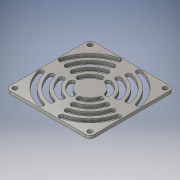
# Autodesk Inventor part: Lüftergitter
Saved by Autodesk Inventor 2016 (Build 200138000, 138)
## iProperties
Created: 2018-05-17
Part Number: Lüftergitter
Material: Stainless Steel
Document SubType Name: Modeling
Designer: Phil Erle
Density: 8 g/cm^3
Appearance: Semi-Polished
Author: Phil Erle
Autodesk Inventor part; units mm, degrees
ref_plane "YZ Plane" through (0, 0, 0) normal (1, 0, 0) x (0, 1, 0)
ref_plane "XZ Plane" through (0, 0, 0) normal (0, 1, 0) x (-1, 0, 0)
ref_plane "XY Plane" through (0, 0, 0) normal (0, 0, 1) x (1, 0, 0)
sketch "Sketch1" plane through (0, 0, 0) normal (0, 0, 1) x (1, 0, 0)
  line L0 (-40, -40) -> (40, -40)
  line L1 (40, -40) -> (40, 40)
  line L2 (40, 40) -> (-40, 40)
  line L3 (-40, 40) -> (-40, -40)
  line L4 (-40, -40) -> (40, 40) construction
  line L5 (40, -40) -> (-40, 40) construction
  point P0 (0, 0)
  dimension "d0" = 80
  dimension "d1" = 80
  constraints: 12 end point, 2 midpoint, 2 parallel, 1 horizontal, 1 perpendicular
  measures "d0" distance of L1.end L2.end
  measures "d1" distance of L0.end L1.end
extrude "Extrusion1" add sketch "Sketch1" along normal blind 3
sketch "Sketch2" plane through (0, 0, 3) normal (0, 0, 1) x (1, 0, 0)
  arc A0 (-9.8351, 36.7052) -> (-36.7052, 9.8351) centre (0, 0) ccw construction
  arc A1 (-10.4822, 39.12) -> (-39.12, 10.4822) centre (0, 0) ccw
  arc A2 (-9.1881, 34.2904) -> (-34.2904, 9.1881) centre (0, 0) ccw
  arc A3 (-9.1881, 34.2904) -> (-10.4822, 39.12) centre (-9.8351, 36.7052) ccw
  arc A4 (-39.12, 10.4822) -> (-34.2904, 9.1881) centre (-36.7052, 9.8351) ccw
  arc A5 (-7.7646, 28.9778) -> (-28.9778, 7.7646) centre (0, 0) ccw construction
  arc A6 (-8.4116, 31.3926) -> (-31.3926, 8.4116) centre (0, 0) ccw
  arc A7 (-7.1175, 26.563) -> (-26.563, 7.1175) centre (0, 0) ccw
  arc A8 (-7.1175, 26.563) -> (-8.4116, 31.3926) centre (-7.7646, 28.9778) ccw
  arc A9 (-31.3926, 8.4116) -> (-26.563, 7.1175) centre (-28.9778, 7.7646) ccw
  arc A10 (-5.694, 21.2504) -> (-21.2504, 5.694) centre (0, 0) ccw construction
  arc A11 (-6.3411, 23.6652) -> (-23.6652, 6.3411) centre (0, 0) ccw
  arc A12 (-5.047, 18.8356) -> (-18.8356, 5.047) centre (0, 0) ccw
  arc A13 (-5.047, 18.8356) -> (-6.3411, 23.6652) centre (-5.694, 21.2504) ccw
  arc A14 (-23.6652, 6.3411) -> (-18.8356, 5.047) centre (-21.2504, 5.694) ccw
  line L0 (0, 0) -> (-62.4866, 0) construction
  line L1 (0, 0) -> (-61.1079, 16.3738) construction
  line L2 (0, 0) -> (0, 46.5462) construction
  line L3 (0, 0) -> (-12.1401, 45.3074) construction
  arc A15 (-3.6235, 13.523) -> (-13.523, 3.6235) centre (0, 0) ccw construction
  arc A16 (-4.2705, 15.9378) -> (-15.9378, 4.2705) centre (0, 0) ccw
  arc A17 (-2.9764, 11.1081) -> (-11.1081, 2.9764) centre (0, 0) ccw
  arc A18 (-2.9764, 11.1081) -> (-4.2705, 15.9378) centre (-3.6235, 13.523) ccw
  arc A19 (-15.9378, 4.2705) -> (-11.1081, 2.9764) centre (-13.523, 3.6235) ccw
  dimension "d4" = 38
  dimension "d5" = 15
  dimension "d6" = 15
  dimension "d7" = 30
  dimension "d8" = 22
  dimension "d9" = 5
  dimension "d10" = 5
  dimension "d11" = 5
  dimension "d12" = 14
  dimension "d13" = 5
  constraints: 40 point on circle, 20 centre point, 16 tangent, 8 end point, 8 point on line, 4 coincident, 1 horizontal, 1 vertical
  measures "d4" radius of A0
  measures "d5" angle of L0 L1
  measures "d6" angle of L3 L2
  measures "d7" radius of A5
  measures "d8" radius of A10
  measures "d9" radial gap between concentric circles of A2 A1
  measures "d10" radial gap between concentric circles of A7 A6
  measures "d11" radial gap between concentric circles of A12 A11
  measures "d12" radius of A15
  measures "d13" diameter of A18
extrude "Extrusion2" cut sketch "Sketch2" against normal blind 3
pattern_circular "Circular Pattern1" count 4 over 360 about axis through (0, 0, -10) along (0, 0, 1) of "Extrusion2"
sketch "Sketch3" plane through (0, 0, 3) normal (0, 0, 1) x (1, 0, 0)
  line L0 (-35.75, -35.75) -> (35.75, -35.75) construction
  line L1 (35.75, -35.75) -> (35.75, 35.75) construction
  line L2 (35.75, 35.75) -> (-35.75, 35.75) construction
  line L3 (-35.75, 35.75) -> (-35.75, -35.75) construction
  line L4 (-35.75, -35.75) -> (35.75, 35.75) construction
  line L5 (35.75, -35.75) -> (-35.75, 35.75) construction
  point P0 (0, 0)
  dimension "d19" = 71.5
  dimension "d20" = 71.5
  constraints: 12 end point, 4 coincident, 2 midpoint, 2 parallel, 1 horizontal, 1 perpendicular
  measures "d19" distance of L2.end L1.end
  measures "d20" distance of L1.end L0.end
hole "Hole1" at (-35.75, 35.75, 3) at (35.75, 35.75, 3) at (35.75, -35.75, 3) at (-35.75, -35.75, 3) direction (0, 0, -1) diameter 4.5 depth 8 tip angle 118 clearance for "Countersunk Flat Head Screw DIN EN ISO 2009" size "M4" standard "DIN"
fillet "Fillet1" radius 4 4 edges at (-40, 40, 1.5) (-40, -40, 1.5) (40, -40, 1.5) (40, 40, 1.5)
body "Solid1"
